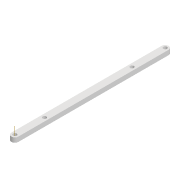
# Autodesk Inventor part: Part_3
Saved by Autodesk Inventor 2022 (Build 260153000, 153)
## iProperties
Created: 2022-04-22
Part Number: Part_3
Material: Generic
Document SubType Name: Modeling
Designer: dell
Density: 1 g/cm^3
Appearance: Default
Author: dell
Autodesk Inventor part; units mm, degrees
ref_plane "YZ Plane" through (0, 0, 0) normal (1, 0, 0) x (0, 1, 0)
ref_plane "XZ Plane" through (0, 0, 0) normal (0, 1, 0) x (-1, 0, 0)
ref_plane "XY Plane" through (0, 0, 0) normal (0, 0, 1) x (1, 0, 0)
sketch "Sketch1" plane through (0, 0, 0) normal (0, 1, 0) x (-1, 0, 0)
  line L0 (0, 0) -> (0, -129.784) construction
  line L1 (3, 0) -> (3, -129.784)
  line L2 (-3, -129.784) -> (-3, 0)
  arc A0 (3, 0) -> (-3, 0) centre (0, 0) ccw
  arc A1 (-3, -129.784) -> (3, -129.784) centre (0, -129.784) ccw
  circle A2 centre (0, 0) radius 1.6
  circle A3 centre (0, -129.784) radius 1.6
  circle A4 centre (0, -25.613) radius 1.6
  circle A5 centre (0, -101.165) radius 1.6
  point P0 (0, -64.892)
  dimension "d0" = 3.2
  dimension "d1" = 3.2
  dimension "d2" = 6
  dimension "d3" = 129.784
  dimension "d4" = 3.2
  dimension "d5" = 25.613
  dimension "d8" = 3.2
  dimension "d9" = 101.165
  constraints: 8 end point, 6 centre point, 4 point on circle, 4 tangent, 2 coincident, 2 point on line, 1 midpoint, 1 parallel, 1 vertical
  measures "d0" diameter of A2
  measures "d1" diameter of A3
  measures "d2" distance between parallel lines of L2 L1
  measures "d3" distance of L0.end L0.start
  measures "d4" diameter of A4
  measures "d5" distance of L0.start A4.centre
  measures "d8" diameter of A5
  measures "d9" distance of L0.start A5.centre
extrude "Extrusion1" add sketch "Sketch1" along normal blind 4
body "Solid1"
